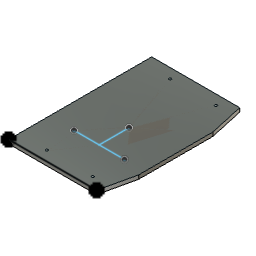
doska v8 (Autodesk Fusion 360 design; units mm, degrees)
Autodesk Fusion 360 part; units mm, degrees
note: some values were not read from the file. Set by a fixed rule: which sketch regions a step uses.
sketch "Sketch1" plane through (0, 0, 0) normal (0, 0, 1) x (1, 0, 0)
  line L0 (125, 90) -> (-125, 90)
  line L1 (-125, 90) -> (-125, -90)
  line L2 (-125, -90) -> (125, -90)
  line L3 (125, -90) -> (125, 90)
  line L4 (125, 90) -> (-125, -90) construction
  line L5 (-125, 90) -> (125, -90) construction
  line L6 (0, 90) -> (-97, 90)
  line L7 (0, 0) -> (0, 90)
  line L8 (0, 90) -> (97, 90)
  line L9 (-97, 90) -> (-97, 77)
  circle A0 centre (-97, 77) radius 1.6
  line L10 (0, 90) -> (-37, 90)
  line L11 (-37, 90) -> (-37, 77)
  circle A1 centre (-37, 77) radius 1.6
  line L12 (97, 90) -> (97, 77)
  line L13 (0, 90) -> (-115, 90)
  line L14 (-115, 90) -> (-125, 44.9959)
  line L15 (-125, 44.9959) -> (-125, 90)
  line L16 (-125, 90) -> (-115, 90)
  line L17 (0, 0) -> (0, -90)
  line L18 (115, 90) -> (125, 44.9959)
  line L19 (125, 44.9959) -> (125, 90)
  line L20 (125, 90) -> (115, 90)
  line L21 (-125, -44.9959) -> (-125, -90)
  line L22 (-125, -90) -> (-115, -90)
  line L23 (125, -44.9959) -> (125, -90)
  line L24 (125, -90) -> (115, -90)
  line L25 (-97, 77) -> (-97, -84)
  line L26 (-97, -84) -> (-97, -90)
  line L27 (-97, -84) -> (-97, -97)
  line L28 (-97, -97) -> (-125.0061, -97)
  line L29 (-125.0061, -97) -> (-125, -90)
  line L30 (-97, -97) -> (125, -97)
  line L31 (125, -97) -> (125, -90)
  line L32 (-37, 77) -> (-37, -84)
  circle A2 centre (-97, -84) radius 1.6
  circle A3 centre (-37, -84) radius 1.6
  circle A4 centre (97, -84) radius 1.6
  circle A5 centre (37, -84) radius 1.6
  circle A6 centre (97, 77) radius 1.6
  circle A7 centre (37, 77) radius 1.6
  line L33 (0, -97) -> (0, 90)
  line L34 (-125.0061, -97) -> (-125.0061, -3.5)
  line L35 (-125.0061, -3.5) -> (125, -3.5)
  line L36 (115, 90) -> (125, 44.9959)
  line L37 (-115, -97) -> (-125, -51.9959)
  line L38 (115, -97) -> (125, -51.9959)
  dimension "d1" = 250
  dimension "d2" = 180
  dimension "d3" = 97
  dimension "d4" = 13
  dimension "d5" = 3.2
  dimension "d6" = 37
  dimension "d7" = 13
  dimension "d8" = 3.2
  dimension "d9" = 115
  dimension "d14" = 161
  dimension "d15" = 13
  dimension "d16" = 161
  dimension "d17" = 3.2
  dimension "d18" = 3.2
  dimension "d19" = 93.5
  constraint perpendicular L0 L1
  constraint parallel L1 L3
  constraint coincident L4 L7.start
  constraint coincident L5 L7.start
  constraint coincident L7.start L17.start
  constraint midpoint L0 L6.start
  constraint parallel L0 L6
  constraint symmetric L6.start L7 L8.start
  constraint perpendicular L0 L9
  constraint coincident L9.end A0.centre
  constraint perpendicular L7 L10
  constraint perpendicular L10 L11
  constraint coincident L11.end A1.centre
  constraint perpendicular L7 L13
  constraint coincident L1 L14.end
  constraint perpendicular L15 L16
  constraint symmetric L0.end L17 L0.start
  constraint symmetric L13.end L17 L18.start
  constraint symmetric L14.end L17 L18.end
  constraint parallel L9 L25
  constraint coincident L2 L26.end
  constraint perpendicular L2 L26
  constraint perpendicular L2 L27
  constraint perpendicular L27 L28
  constraint perpendicular L27 L30
  constraint perpendicular L24 L31
  constraint coincident L25.end L26.start
  constraint coincident L32.end A3.centre
  constraint symmetric A0 L17 A6
  constraint symmetric A1 L17 A7
  constraint symmetric L17 A2 A4
  constraint symmetric L17 A3 A5
  constraint coincident L30 L33.start
  constraint perpendicular L10 L33
  constraint perpendicular L22 L34
  constraint coincident L3 L35.end
  constraint perpendicular L3 L35
  constraint symmetric L13.end L33 L18.start
  constraint symmetric L14.end L33 L18.end
  constraint symmetric L13.end L35 L37.start
  constraint symmetric L14.end L35 L37.end
  constraint symmetric L17 L37.start L38.start
  constraint symmetric L17 L37.end L38.end
  measures "d1" distance of L1.end L2.end
  measures "d2" distance of L0.end L1.end
  measures "d3" distance of L6.start L6.end
  measures "d4" distance of L6.end L9.end
  measures "d5" diameter of A0
  measures "d6" distance of L6.start L10.end
  measures "d7" distance of L10.end L11.end
  measures "d8" diameter of A1
  measures "d9" distance of L6.start L13.end
  measures "d14" distance of L9.end L25.end
  measures "d15" distance of L25.end L27.end
  measures "d16" distance of L11.end L32.end
  measures "d17" diameter of A2
  measures "d18" diameter of A3
  measures "d19" distance of L28.end L34.end
extrude "Extrude3" add sketch "Sketch1" against normal blind 5 contours L0 L3 L7 L8 L17 L18 L33 L35 L36 | L2 L3 L17 L23 L24 L33 L35 L38 | L2 L24 L30 L33 L38 | A4 | A5 | A6 | A7
extrude "Extrude4" cut sketch "Sketch1" against normal blind 10 contours L11 A1 L32 | L9 A0 L25 | L25 L26 L27 A2 | A4 | A5 | A6 | A7 picked at (-36.3624, 76.1483) picked at (-96.2477, 77.7523) picked at (-96.2477, -84.7523)
sketch "Sketch3" plane through (0, 0, 0) normal (0, 0, 1) x (-1, 0, 0)
  circle A0 centre (-97, 84) radius 1.6
  circle A1 centre (-97, -77) radius 1.6
  circle A2 centre (-37, 84) radius 1.6
  circle A3 centre (-37, -77) radius 1.6
  line L0 (0, 97) -> (-115, 97)
  line L1 (-115, 97) -> (-125, 51.9959)
  line L2 (-125, 51.9959) -> (-125, -44.9959)
  line L3 (-125, -44.9959) -> (-115, -90)
  line L4 (-115, -90) -> (0, -90)
  line L5 (0, -90) -> (0, 97)
  line L6 (0, 97) -> (-115, 97)
  line L7 (-32.4552, 44.0647) -> (-98.4552, 44.0647)
  circle A4 centre (-32.4552, 44.0647) radius 1.25
  circle A5 centre (-98.4552, 44.0647) radius 1.25
  line L8 (-65.4552, 44.0647) -> (-65.4552, 5.0647)
  circle A6 centre (-65.4552, 5.0647) radius 1.25
  dimension "d28" = 115
  dimension "d29" = 60
  dimension "d30" = 66
  dimension "d31" = 2.5
  dimension "d32" = 2.5
  dimension "d33" = 39
  dimension "d34" = 2.5
  constraint coincident L0.start L5.end
  constraint coincident L0.end L1.start
  constraint horizontal L7
  constraint coincident L7.start A4.centre
  constraint coincident L7.end A5.centre
  constraint midpoint L7 L8.start
  constraint perpendicular L7 L8
  constraint coincident L8.end A6.centre
  measures "d28" distance of L0.start L0.end
  measures "d29" distance of A0.centre A2.centre
  measures "d30" distance of L7.start L7.end
  measures "d31" diameter of A4
  measures "d32" diameter of A5
  measures "d33" distance of L8.start L8.end
  measures "d34" diameter of A6
extrude "Extrude6" cut sketch "Sketch3" against normal blind 30 contours A4 | A5 | A6
